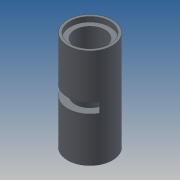
# Autodesk Inventor part: 62462-LtBluishGray
Saved by Autodesk Inventor 2022.2 (Build 262287000, 287)
## iProperties
Created: 2014-07-31
Part Number: 62462-LtBluishGray
Material: ABS Plastic
Document SubType Name: Modeling
Designer: D. Kohfeld
Mass: 0.335775 g
Surface Area: 6.7306 cm^2
Volume: 0.316769 cm^3
Density: 1.06 g/cm^3
Appearance: LtBluishGray
Author: D. Kohfeld
Autodesk Inventor part; units mm, degrees
ref_plane "YZ Plane" through (0, 0, 0) normal (1, 0, 0) x (0, 1, 0)
ref_plane "XZ Plane" through (0, 0, 0) normal (0, 1, 0) x (-1, 0, 0)
ref_plane "XY Plane" through (0, 0, 0) normal (0, 0, 1) x (1, 0, 0)
sketch "Sketch2" plane through (0, 0, 0) normal (0, 0, 1) x (1, 0, 0)
  line L0 (0, -11.2) -> (0, 11.2) projected
  line L1 (-3.6, 8) -> (-3.6, -8)
  line L2 (-3.6, -8) -> (-3.2, -8)
  line L3 (-3.2, -8) -> (-3.2, -7.2)
  line L4 (-3.2, -7.2) -> (-2.4, -7.2)
  line L5 (-2.4, -7.2) -> (-2.4, -0.8)
  line L6 (-2.4, -0.8) -> (-3.2, -0.8)
  line L7 (-3.2, -0.8) -> (-3.2, 0.8)
  line L8 (-3.2, 0.8) -> (-2.4, 0.8)
  line L9 (-2.4, 0.8) -> (-2.4, 7.2)
  line L10 (-2.4, 7.2) -> (-3.2, 7.2)
  line L11 (-3.2, 7.2) -> (-3.2, 8)
  line L12 (-3.2, 8) -> (-3.6, 8)
  point P0 (0, 0)
  point P1 (-3.2, 0)
  dimension "d0" = 16
  dimension "d1" = 6.4
  dimension "d2" = 7.2
  dimension "d3" = 4.8
  dimension "d4" = 0.8
  dimension "d5" = 1.6
  constraints: 24 end point, 10 parallel, 5 equal length, 1 horizontal, 1 horizontal alignment, 1 midpoint, 1 perpendicular
  measures "d0" distance of L1.start L1.end
  measures "d1" diameter of L11 L0
  measures "d2" diameter of L1 L0
  measures "d3" diameter of L9 L0
  measures "d4" distance between parallel lines of L10 L12
  measures "d5" distance between parallel lines of L6 L8
revolve "Revolution1" add sketch "Sketch2" angle 360 about axis through (0, -10, 0) along (0, 1, 0)
sketch "Sketch3" plane through (0, 0, 0) normal (0, 1, 0) x (-1, 0, 0)
  circle A0 centre (0, 0) radius 3.2 projected
  circle A1 centre (0, 0) radius 3.6 projected
  line L0 (-3.2, 0) -> (-3.2, 1.6492)
  line L1 (3.2, 0) -> (3.2, 1.6492)
  constraints: 4 end point, 4 point on circle, 2 tangent, 1 parallel, 1 vertical
extrude "Extrusion1" cut sketch "Sketch3" along normal up to surface (1.6 mm away) from surface at -0.8 contours A0 L0 A1 L1 picked at (-0.1286, 3.4412)
equation "\"d0\" = 2 * lu"
equation "\"d1\" = tsd"
equation "\"d2\" = tlad"
equation "\"d3\" = tpd"
equation "\"d4\" = tsl"
equation "\"d5\" = 2 * tsl"
equation "\"lu\" = 8"
equation "\"tsd\" = 6.4"
equation "\"tlad\" = 7.2"
equation "\"tpd\" = 4.8"
equation "\"tsl\" = 0.8"
body "Solid1"
